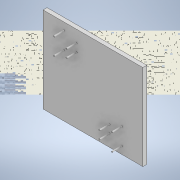
# Autodesk Inventor part: Placa
Saved by Autodesk Inventor 2022 (Build 260153000, 153)
## iProperties
Created: 2022-11-13
Part Number: Placa
Material: Genérico
Document SubType Name: Modeling
Designer: Usuario
Density: 1 g/cm^3
Appearance: Valor por defecto
Author: Usuario
Autodesk Inventor part; units mm, degrees
ref_plane "YZ Plane" through (0, 0, 0) normal (1, 0, 0) x (0, 1, 0)
ref_plane "XZ Plane" through (0, 0, 0) normal (0, 1, 0) x (-1, 0, 0)
ref_plane "XY Plane" through (0, 0, 0) normal (0, 0, 1) x (1, 0, 0)
sketch "Boceto1" plane through (0, 0, 0) normal (0, 0, 1) x (1, 0, 0)
  line L0 (-250, -215) -> (250, -215)
  line L1 (250, -215) -> (250, 215)
  line L2 (250, 215) -> (-250, 215)
  line L3 (-250, 215) -> (-250, -215)
  line L4 (-250, -215) -> (250, 215) construction
  line L5 (250, -215) -> (-250, 215) construction
  point P0 (0, 0)
  dimension "d0" = 500
  dimension "d1" = 430
  constraints: 12 end point, 2 midpoint, 2 parallel, 1 horizontal, 1 perpendicular
  measures "d0" distance of L2.end L1.end
  measures "d1" distance of L1.end L0.end
extrude "Extrusión1" add sketch "Boceto1" along normal blind 20
sketch "Boceto7" plane through (0, 0, 20) normal (0, 0, 1) x (1, 0, 0)
  line L0 (-135.0434, 135.4344) -> (-155.0434, 135.4344)
  line L1 (-155.0434, 170.4344) -> (-155.0434, 100.4344)
  line L2 (-145.0434, 135.4344) -> (-145.0434, 185.4344)
  line L3 (-70.0434, 185.4344) -> (-200.0434, 185.4344)
  line L4 (-145.0434, 170.4344) -> (-145.0434, 185.4344)
  line L5 (-145.0434, 185.4344) -> (-145.0434, 177.9344)
  line L6 (-145.0434, 135.4344) -> (-70.0434, 135.4344)
  line L7 (-70.0434, 85.4344) -> (-70.0434, 185.4344)
  line L8 (-95.0434, 170.4344) -> (-95.0434, 100.4344)
  line L9 (-95.0434, 135.4344) -> (-70.0434, 135.4344)
  line L10 (-82.5434, 135.4344) -> (-82.5434, 155.4344)
  circle A0 centre (-145.0434, 177.9344) radius 3
  circle A1 centre (-82.5434, 155.4344) radius 3
  circle A2 centre (-145.0434, 92.9344) radius 3
  circle A3 centre (-82.5434, 115.4344) radius 3
  line L11 (-250, 215) -> (-250, -215) projected
  line L12 (-250, 215) -> (-200, 215)
  line L13 (-200, 215) -> (-200, 185)
  line L14 (-250, 0) -> (0, 0)
  line L15 (250, -215) -> (-250, -215)
  line L16 (135.0434, -135.4344) -> (155.0434, -135.4344)
  line L17 (155.0434, -170.4344) -> (155.0434, -100.4344)
  line L18 (145.0434, -135.4344) -> (70.0434, -135.4344)
  line L19 (-250, -215) -> (250, -215)
  line L20 (70.0434, -185.4344) -> (200.0434, -185.4344)
  line L21 (145.0434, -185.4344) -> (145.0434, -177.9344)
  line L22 (145.0434, -170.4344) -> (145.0434, -185.4344)
  circle A4 centre (145.0434, -177.9344) radius 3
  circle A5 centre (145.0434, -92.9344) radius 3
  line L23 (200, -215) -> (200, -185)
  line L24 (145.0434, -135.4344) -> (145.0434, -185.4344)
  line L25 (250, -215) -> (200, -215)
  line L26 (95.0434, -170.4344) -> (95.0434, -100.4344)
  line L27 (70.0434, -85.4344) -> (70.0434, -185.4344)
  circle A6 centre (82.5434, -115.4344) radius 3
  line L28 (82.5434, -135.4344) -> (82.5434, -155.4344)
  circle A7 centre (82.5434, -155.4344) radius 3
  line L29 (95.0434, -135.4344) -> (70.0434, -135.4344)
  point P0 (250, 215)
  dimension "d22" = 20
  dimension "d23" = 6
  dimension "d24" = 6
  dimension "d25" = 50
  dimension "d26" = 30
  constraints: 58 end point, 8 centre point, 7 midpoint, 5 point on line, 4 coincident, 2 symmetric about line, 1 horizontal, 1 perpendicular
  measures "d22" distance of L10.start L10.end
  measures "d23" diameter of A0
  measures "d24" diameter of A1
  measures "d25" distance of L11.start L12.end
  measures "d26" distance of L12.end L13.end
extrude "Extrusión7" add sketch "Boceto7" along normal blind 50 contours A1 | A0 L2 | L2 A0 | A2 | A3
extrude "Extrusión8" add sketch "Boceto7" along normal blind 50 contours A7 | A4 L22 L21 | L21 L22 A4 | A5 | A6
